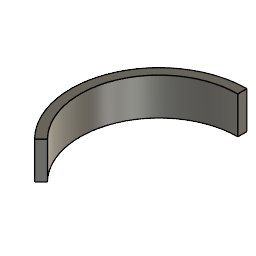
RingCase (Autodesk Fusion 360 archive; units mm, degrees)
design "GrepowBattery"
Autodesk Fusion 360 part; units mm, degrees
sketch "Sketch1" plane through (0, 0, 0) normal (0, 0, 1) x (1, 0, 0)
  arc A0 (0, 14.1125) -> (-7.868, -11.7157) centre (0, 0) ccw
  line L0 (0, 0) -> (0, 14.1125) construction
  line L1 (0, 0) -> (-7.868, -11.7157) construction
  dimension "d1" = 14.1125
  dimension "d2" = 146.115
  constraint coincident A0.centre L0.start
  measures "d1" radius of A0
  measures "d2" angle of L0 L1
sketch "Sketch2" plane through (0, 0, 0) normal (1, 0, 0) x (0, 1, 0)
sketch "Sketch3" plane through (0, 0, 0) normal (1, 0, 0) x (0, 1, 0)
  line L0 (13.3068, 3.26) -> (14.9182, 3.26)
  line L1 (14.9182, 3.26) -> (14.9182, -3.26)
  line L2 (14.9182, -3.26) -> (13.3068, -3.26)
  line L3 (13.3068, -3.26) -> (13.3068, 3.26)
  line L4 (13.3068, 3.26) -> (14.9182, -3.26) construction
  line L5 (14.9182, 3.26) -> (13.3068, -3.26) construction
  point P0 (14.1125, 0)
  dimension "d3" = 6.52
  constraint horizontal L0
  constraint perpendicular L0 L1
  constraint parallel L0 L2
  constraint parallel L1 L3
  constraint coincident L4 P0
  constraint coincident L5 P0
  measures "d3" distance of L0.end L1.end
sketch "Sketch4" plane through (0, 0, 0) normal (0, 0, 1) x (1, 0, 0)
  arc A0 (0, 14.625) -> (-10.3847, -10.298) centre (0, 0) ccw
  line L0 (0, 0) -> (0, 14.625) construction
  line L1 (0, 0) -> (-10.3847, -10.298) construction
  dimension "d10" = 14.625
  dimension "d11" = 134.76
  constraint coincident A0.centre L0.start
  measures "d10" radius of A0
  measures "d11" angle of L0 L1
sketch "Sketch5" plane through (0, 0, 0) normal (1, 0, 0) x (0, 1, 0)
  line L0 (13.8198, 3.26) -> (15.4302, 3.26)
  line L1 (15.4302, 3.26) -> (15.4302, -3.26)
  line L2 (15.4302, -3.26) -> (13.8198, -3.26)
  line L3 (13.8198, -3.26) -> (13.8198, 3.26)
  line L4 (13.8198, 3.26) -> (15.4302, -3.26) construction
  line L5 (15.4302, 3.26) -> (13.8198, -3.26) construction
  point P0 (14.625, 0)
  dimension "d12" = 6.52
  constraint horizontal L0
  constraint perpendicular L0 L1
  constraint parallel L0 L2
  constraint parallel L1 L3
  constraint coincident L4 P0
  constraint coincident L5 P0
  measures "d12" distance of L0.end L1.end
sweep "Sweep2" add profiles "Sketch5" path "Sketch4" along A0 section 1

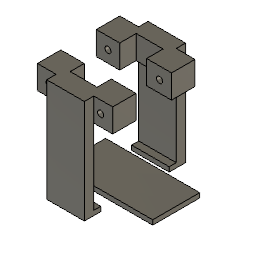
design "Holder"
Autodesk Fusion 360 part; units mm, degrees
sketch "Sketch1" plane through (0, 0, 0) normal (0, 0, 1) x (1, 0, 0)
  line L0 (0, 0) -> (5.7, 0)
  line L1 (5.7, 0) -> (5.7, 6.5)
  line L2 (5.7, 6.5) -> (0, 6.5)
  line L3 (0, 6.5) -> (0, 0)
  line L4 (-2, 8) -> (8, 8)
  line L5 (8, 8) -> (8, -2)
  line L6 (8, -2) -> (-2, -2)
  line L7 (-2, -2) -> (-2, 8)
  dimension "d1" = 5.7
  dimension "d2" = 6.5
  constraint horizontal L0
  constraint vertical L1
  constraint horizontal L2
  constraint vertical L3
  constraint coincident L0.start L3.end
  constraint horizontal L4
  constraint vertical L5
  constraint horizontal L6
  constraint vertical L7
  measures "d1" distance of L0.start L0.end
  measures "d2" distance of L0.start L2.end
extrude "Extrude1" add sketch "Sketch1" along normal blind 5 makes body 1
move_body "Move1" bodies 1 to x (1, 0, 0) y (0, 1, 0) z (0, 0, 1) at (0, 0, 15)
sketch "Sketch2" plane through (0, 0, 0) normal (0, 0, 1) x (1, 0, 0)
  line L0 (-2, 8) -> (18, 8)
  line L1 (18, 8) -> (18, -2)
  line L2 (18, -2) -> (-2, -2)
  line L3 (-2, -2) -> (-2, 8)
  dimension "d5" = 20
  dimension "d6" = 10
  constraint horizontal L0
  constraint vertical L1
  constraint horizontal L2
  constraint vertical L3
  measures "d5" distance of L0.start L0.end
  measures "d6" distance of L0.start L2.end
extrude "Extrude2" add sketch "Sketch2" against normal blind 1 separate body makes body 2
sketch "Sketch3" plane through (0, -2, 0) normal (0, -1, 0) x (1, 0, 0)
  line L0 (-2, 15) -> (8, 15)
  line L1 (8, 15) -> (8, 20)
  line L2 (8, 20) -> (-2, 20)
  line L3 (-2, 20) -> (-2, 15)
  line L4 (0, 20) -> (4, 20)
  line L5 (4, 20) -> (4, 15)
  line L6 (4, 15) -> (0, 15)
  line L7 (0, 15) -> (0, 20)
  dimension "d9" = 4
  constraint horizontal L4
  constraint vertical L5
  constraint horizontal L6
  constraint vertical L7
  constraint coincident L2 L4.start
  measures "d9" distance of L4.start L4.end
extrude "Extrude3" add sketch "Sketch3" along normal blind 2 contours L0 L2 L4 L5 L6 L7 bodies 1
sketch "Sketch4" plane through (0, 8, 0) normal (0, 1, 0) x (-1, 0, 0)
  line L0 (-8, 15) -> (2, 15)
  line L1 (2, 15) -> (2, 20)
  line L2 (2, 20) -> (-8, 20)
  line L3 (-8, 20) -> (-8, 15)
  line L4 (-4, 20) -> (0, 20)
  line L5 (0, 20) -> (0, 15)
  line L6 (0, 15) -> (-4, 15)
  line L7 (-4, 15) -> (-4, 20)
  dimension "d12" = 4
  constraint horizontal L4
  constraint vertical L5
  constraint horizontal L6
  constraint vertical L7
  constraint coincident L2 L4.start
  measures "d12" distance of L4.start L4.end
extrude "Extrude4" add sketch "Sketch4" along normal blind 2 contours L0 L2 L4 L5 L6 L7 bodies 1
sketch "Sketch5" plane through (0, 0, 15) normal (0, 0, -1) x (1, 0, 0)
  line L0 (0, -6.5) -> (0, 0)
  line L1 (0, 0) -> (5.7, 0)
  line L2 (5.7, 0) -> (5.7, -6.5)
  line L3 (5.7, -6.5) -> (0, -6.5)
  line L4 (8, 2) -> (4, 2)
  line L5 (4, 2) -> (4, 4)
  line L6 (4, 4) -> (0, 4)
  line L7 (0, 4) -> (0, 2)
  line L8 (0, 2) -> (-2, 2)
  line L9 (-2, 2) -> (-2, -8)
  line L10 (-2, -8) -> (0, -8)
  line L11 (0, -8) -> (0, -10)
  line L12 (0, -10) -> (4, -10)
  line L13 (4, -10) -> (4, -8)
  line L14 (4, -8) -> (8, -8)
  line L15 (8, -8) -> (8, 2)
  line L16 (4, -8) -> (0, -8)
  line L17 (0, -8) -> (0, -10)
  line L18 (0, -10) -> (4, -10)
  line L19 (4, -10) -> (4, -8)
  line L20 (4, 4) -> (0, 4)
  line L21 (0, 4) -> (0, 2)
  line L22 (0, 2) -> (4, 2)
  line L23 (4, 2) -> (4, 4)
  constraint horizontal L16
  constraint vertical L17
  constraint horizontal L18
  constraint vertical L19
  constraint coincident L11.end L12.start
  constraint coincident L13.end L14.start
  constraint horizontal L20
  constraint vertical L21
  constraint horizontal L22
  constraint vertical L23
  constraint coincident L7.end L8.start
  constraint coincident L5.end L6.start
extrude "Extrude5" add sketch "Sketch5" along normal blind 17 contours L5 L6 L7 L20 L21 L22 L23 | L11 L12 L13 L16 L17 L18 L19 bodies 1
sketch "Sketch6" plane through (0, 8, 0) normal (0, -1, 0) x (1, 0, 0)
  line L0 (4, 15) -> (0, 15)
  line L1 (0, 15) -> (0, -2)
  line L2 (0, -2) -> (4, -2)
  line L3 (4, -2) -> (4, 15)
  line L4 (0, -2) -> (4, -2)
  line L5 (4, -2) -> (4, -1)
  line L6 (4, -1) -> (0, -1)
  line L7 (0, -1) -> (0, -2)
  dimension "d17" = 1
  constraint horizontal L4
  constraint vertical L5
  constraint horizontal L6
  constraint vertical L7
  constraint coincident L1.end L2.start
  measures "d17" distance of L1.end L6.end
extrude "Extrude6" add sketch "Sketch6" along normal blind 2 contours L1 L2 L3 L4 L5 L6 L7 bodies 1
sketch "Sketch7" plane through (0, -2, 0) normal (0, 1, 0) x (-1, 0, 0)
  line L0 (0, 15) -> (-4, 15)
  line L1 (-4, 15) -> (-4, -2)
  line L2 (-4, -2) -> (0, -2)
  line L3 (0, -2) -> (0, 15)
  line L4 (-4, -2) -> (0, -2)
  line L5 (0, -2) -> (0, -1)
  line L6 (0, -1) -> (-4, -1)
  line L7 (-4, -1) -> (-4, -2)
  dimension "d20" = 1
  constraint horizontal L4
  constraint vertical L5
  constraint horizontal L6
  constraint vertical L7
  constraint coincident L1.end L2.start
  measures "d20" distance of L1.end L6.end
extrude "Extrude7" add sketch "Sketch7" along normal blind 2 contours L1 L2 L3 L4 L5 L6 L7 bodies 1
move_body "Move2" bodies 1 to x (1, 0, 0) y (0, 1, 0) z (0, 0, 1) at (-3, -3, 0)
extrude "Extrude8" add 1 faces at (5, 1.6667, 16.6667) along direction (1, 0, 0) blind 3 on bodies 1 bodies 1
extrude "Extrude9" add 1 faces at (-5, -1.6667, 16.6667) along direction (-1, 0, 0) blind 3 on bodies 1 bodies 1
hole "Hole1" at (5.4307, 5, 17.4525) direction (0, -1, 0) diameter 1.3 depth 11 tip angle 118 counterbore diameter 3 counterbore depth 1.5 bodies 1
hole "Hole2" at (-5.5, 5, 17.5) direction (0, -1, 0) diameter 1.3 depth 11 tip angle 118 counterbore diameter 3 counterbore depth 1.5 bodies 1
split "Split1" by plane through (0, 0, 0) normal (0, 1, 0) bodies 1 makes body 3 at (-1.6667, 7, 5.3333)
move_body "Move3" bodies 1 to x (1, 0, 0) y (0, 1, 0) z (0, 0, 1) at (0, -7.5, 0)
extrude "Extrude10" add 2 faces at (1, 6.3333, 11) (1, -13.8333, 11) along direction (1, 0, 0) blind 3 on bodies 1 3 bodies 3 1
extrude "Extrude11" add 2 faces at (-3, 6.3333, 11) (-3, -13.8333, 11) along direction (-1, 0, 0) blind 1 on bodies 1 3 bodies 3 1
extrude "Extrude12" cut 1 faces at (1.3333, 3, -1.3333) along direction (0, 1, 0) blind 0.5 on bodies 3 bodies 3
extrude "Extrude13" cut 1 faces at (-1.3333, -10.5, -1.6667) along direction (0, -1, 0) blind 0.5 on bodies 1 bodies 1
move_body "Move4" bodies 2 to x (1, 0, 0) y (0, 1, 0) z (0, 0, 1) at (-5, -7, 0)
